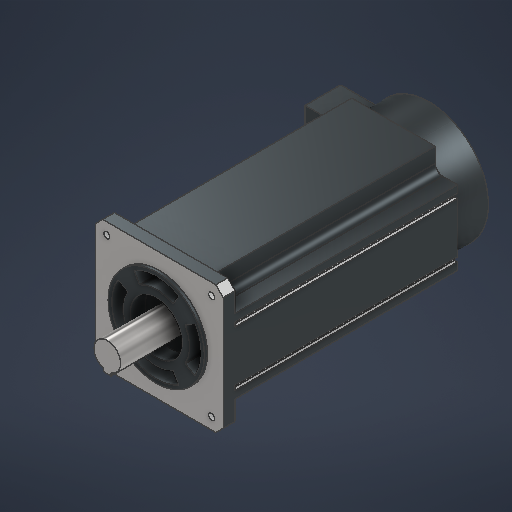
# Autodesk Inventor part: SERVOMOTOR-1KW
Saved by Autodesk Inventor 2025.3 (Build 293356030, 356C)
## iProperties
Created: 2025-09-01
Part Number: SERVOMOTOR-1KW
Material: Generic
Document SubType Name: Modeling
Designer: lstk1ng
Density: 1 g/cm^3
Appearance: Default
Author: lstk1ng
Autodesk Inventor part; units mm, degrees
ref_plane "YZ Plane" through (0, 0, 0) normal (1, 0, 0) x (0, 1, 0)
ref_plane "XZ Plane" through (0, 0, 0) normal (0, 1, 0) x (-1, 0, 0)
ref_plane "XY Plane" through (0, 0, 0) normal (0, 0, 1) x (1, 0, 0)
sketch "Sketch1" plane through (0, 0, 0) normal (0, 0, 1) x (1, 0, 0)
  line L0 (-38.15, 43.15) -> (38.15, 43.15)
  line L1 (43.15, 38.15) -> (43.15, -38.15)
  line L2 (38.15, -43.15) -> (-38.15, -43.15)
  line L3 (-43.15, -38.15) -> (-43.15, 38.15)
  circle A0 centre (0, 0) radius 32.5
  line L4 (-43.15, 38.15) -> (-38.15, 43.15)
  line L5 (38.15, 43.15) -> (43.15, 38.15)
  line L6 (-43.15, -38.15) -> (-38.15, -43.15)
  line L7 (38.15, -43.15) -> (43.15, -38.15)
  point P0 (-43.15, 43.15)
  point P1 (43.15, -43.15)
  point P2 (43.15, 43.15)
  point P3 (-43.15, -43.15)
  point P4 (-43.15, 0)
  dimension "d0" = 86.3
  dimension "d1" = 86.3
  dimension "d2" = 65
  dimension "d3" = 5
  dimension "d4" = 5
  dimension "d5" = 5
  dimension "d6" = 5
  dimension "d7" = 5
  dimension "d8" = 5
  dimension "d9" = 5
  dimension "d10" = 5
  constraints: 16 end point, 8 point on line, 2 parallel, 1 centre point, 1 coincident, 1 horizontal, 1 horizontal alignment, 1 midpoint, 1 perpendicular
  measures "d0" distance of point (43.15, -43.15) point (-43.15, -43.15)
  measures "d1" distance of point (43.15, 43.15) point (43.15, -43.15)
  measures "d2" diameter of A0
  measures "d3" distance of L3.end point (-43.15, 43.15)
  measures "d4" distance of L0.start point (-43.15, 43.15)
  measures "d5" distance of L0.end point (43.15, 43.15)
  measures "d6" distance of L1.start point (43.15, 43.15)
  measures "d7" distance of L3.start point (-43.15, -43.15)
  measures "d8" distance of L2.end point (-43.15, -43.15)
  measures "d9" distance of L2.start point (43.15, -43.15)
  measures "d10" distance of L1.end point (43.15, -43.15)
extrude "Extrusion1" add sketch "Sketch1" along normal blind 8
sketch "Sketch2" plane through (0, 0, 0) normal (0, 0, 1) x (1, 0, 0)
  circle A0 centre (0, 0) radius 32.5
  line L0 (11.25, 19.4856) -> (15, 25.9808)
  line L1 (0, 0) -> (30, 0) construction
  line L2 (-11.25, 19.4856) -> (-15, 25.9808)
  line L3 (0, 0) -> (30, 0) construction
  line L4 (-19.4856, -11.25) -> (-25.9808, -15)
  line L5 (-19.4856, 11.25) -> (-25.9808, 15)
  line L6 (11.25, -19.4856) -> (15, -25.9808)
  line L7 (-11.25, -19.4856) -> (-15, -25.9808)
  line L8 (19.4856, 11.25) -> (25.9808, 15)
  line L9 (19.4856, -11.25) -> (25.9808, -15)
  arc A1 (15, 25.9808) -> (-15, 25.9808) centre (0, 0) ccw
  arc A2 (25.9808, -15) -> (25.9808, 15) centre (0, 0) ccw
  arc A3 (-25.9808, 15) -> (-25.9808, -15) centre (0, 0) ccw
  arc A4 (-15, -25.9808) -> (15, -25.9808) centre (0, 0) ccw
  circle A5 centre (0, 0) radius 17.5
  arc A6 (-19.4856, 11.25) -> (-19.4856, -11.25) centre (0, 0) ccw
  arc A7 (-11.25, -19.4856) -> (11.25, -19.4856) centre (0, 0) ccw
  arc A8 (19.4856, -11.25) -> (19.4856, 11.25) centre (0, 0) ccw
  arc A9 (11.25, 19.4856) -> (-11.25, 19.4856) centre (0, 0) ccw
  dimension "d15" = 60
  dimension "d16" = 120
  dimension "d19" = 360
  dimension "d21" = 35
  constraints: 20 end point, 16 point on circle, 10 centre point, 4 coincident, 2 horizontal, 25 other
  measures "d15" angle of L1 L0
  measures "d16" angle of L3 L2
  measures "d21" diameter of A5
extrude "Extrusion2" add sketch "Sketch2" along normal blind 10
sketch "Sketch3" plane through (0, 0, 0) normal (0, 0, -1) x (-1, 0, 0)
  line L0 (-28.15, 40) -> (28.15, 40)
  line L1 (43.15, 25) -> (43.15, -25)
  line L2 (28.15, -40) -> (-28.15, -40)
  line L3 (-43.15, -25) -> (-43.15, 25)
  line L4 (-43.15, 40) -> (43.15, -40) construction
  line L5 (43.15, 40) -> (-43.15, -40) construction
  line L6 (-43.15, 25) -> (-28.15, 25)
  line L7 (-28.15, 25) -> (-28.15, 40)
  line L8 (28.15, 40) -> (28.15, 25)
  line L9 (28.15, 25) -> (43.15, 25)
  line L10 (-11.6946, 0) -> (10.241, 0) construction
  line L11 (-43.15, -25) -> (-28.15, -25)
  line L12 (-28.15, -25) -> (-28.15, -40)
  line L13 (28.15, -40) -> (28.15, -25)
  line L14 (28.15, -25) -> (43.15, -25)
  point P0 (0, 0)
  constraints: 30 end point, 6 symmetric about line, 3 perpendicular, 2 horizontal, 2 midpoint, 2 parallel
extrude "Extrusion3" add sketch "Sketch3" along normal blind 150
fillet "Fillet1" radius 5 4 edges at (28.15, 25, -75) (-28.15, 25, -75) (-28.15, -25, -75) (28.15, -25, -75)
sketch "Sketch4" plane through (0, 0, -150) normal (0, 0, -1) x (-1, 0, 0)
  arc A0 (34.641, 20) -> (34.641, -20) centre (0, 0) ccw
  line L0 (34.641, 20) -> (59.641, 20)
  line L1 (59.641, 20) -> (59.641, -20)
  line L2 (59.641, -20) -> (34.641, -20)
  dimension "d34" = 25
  dimension "d35" = 40
  constraints: 6 end point, 2 perpendicular, 2 point on circle, 1 centre point, 1 coincident, 1 horizontal
  measures "d34" distance of L0.start L0.end
  measures "d35" distance of L0.end L1.end
extrude "Extrusion4" add sketch "Sketch4" along normal blind 24
sketch "Sketch5" plane through (-43.15, -38.15, 8) normal (-1, 0, 0) x (0, 0, 1)
  line L0 (-158, 12.5091) -> (-158, 63.7909) projected
  line L1 (-158, 18.15) -> (-8, 18.15)
  line L2 (-8, 18.15) -> (-8, 21.15)
  line L3 (-8, 21.15) -> (-158, 21.15)
  line L4 (-158, 21.15) -> (-158, 18.15)
  line L5 (-8, 13.15) -> (-158, 13.15) projected
  line L6 (-158, 58.15) -> (-8, 58.15)
  line L7 (-8, 58.15) -> (-8, 55.15)
  line L8 (-8, 55.15) -> (-158, 55.15)
  line L9 (-158, 55.15) -> (-158, 58.15)
  line L10 (-8, 63.15) -> (-158, 63.15) projected
  point P0 (-8, 38.15)
  dimension "d38" = 3
  dimension "d39" = 5
  dimension "d40" = 3
  dimension "d41" = 5
  constraints: 16 end point, 4 parallel, 2 horizontal, 2 perpendicular, 2 point on line
  measures "d38" distance of L2.end L1.end
  measures "d39" distance between parallel lines of L5 L1
  measures "d40" distance of L6.end L7.end
  measures "d41" distance between parallel lines of L10 L6
extrude "Extrusion5" cut sketch "Sketch5" against normal blind 2
mirror "Mirror1" about plane through (0, 0, 0) normal (1, 0, 0) of "Extrusion5"
sketch "Sketch6" plane through (0, 0, 0) normal (0, 0, 1) x (1, 0, 0)
  arc A0 (2.5, -8.6458) -> (-2.5, -8.6458) centre (0, 0) ccw
  line L0 (0, -9) -> (0, -8) construction
  line L1 (0, -8) -> (-2.5, -8) construction
  line L2 (-2.5, -8) -> (0, -8) construction
  line L3 (2.5, -8) -> (2.5, -10.5)
  line L4 (2.5, -10.5) -> (-2.5, -10.5)
  line L5 (-2.5, -10.5) -> (-2.5, -8)
  dimension "d44" = 18
  dimension "d45" = 1
  dimension "d46" = 2.5
  dimension "d47" = 5
  dimension "d48" = 2.5
  constraints: 12 end point, 2 horizontal, 2 parallel, 2 point on circle, 2 point on line, 1 centre point, 1 coincident, 1 perpendicular, 1 vertical
  measures "d44" diameter of A0
  measures "d45" distance of L0.end L0.start
  measures "d46" distance of L0.end L1.end
  measures "d47" distance of L3.end L4.end
  measures "d48" distance of L3.start L3.end
extrude "Extrusion6" add sketch "Sketch6" along normal blind 43
sketch "Sketch7" plane through (0, 0, 8) normal (0, 0, 1) x (1, 0, 0)
  circle A0 centre (0, 0) radius 50 construction
  line L0 (-43.15, -43.15) -> (43.15, -43.15) construction
  line L1 (43.15, -43.15) -> (43.15, 43.15) construction
  line L2 (43.15, 43.15) -> (-43.15, 43.15) construction
  line L3 (-43.15, 43.15) -> (-43.15, -43.15) construction
  line L4 (-43.15, -43.15) -> (43.15, 43.15) construction
  line L5 (43.15, -43.15) -> (-43.15, 43.15) construction
  circle A1 centre (35.3553, 35.3553) radius 2.05
  circle A2 centre (35.3553, -35.3553) radius 2.05
  circle A3 centre (-35.3553, 35.3553) radius 2.05
  circle A4 centre (-35.3553, -35.3553) radius 2.05
  dimension "d51" = 100
  dimension "d52" = 4.1
  dimension "d53" = 4.1
  dimension "d54" = 4.1
  dimension "d55" = 4.1
  constraints: 12 end point, 5 centre point, 4 point on circle, 4 point on line, 2 midpoint, 2 parallel, 1 coincident, 1 horizontal, 1 perpendicular
  measures "d51" diameter of A0
  measures "d52" diameter of A1
  measures "d53" diameter of A2
  measures "d54" diameter of A3
  measures "d55" diameter of A4
extrude "Extrusion7" cut sketch "Sketch7" against normal up to surface (8 mm away)
equation "\"d4\" = d3"
equation "\"d5\" = d3"
equation "\"d6\" = d5"
equation "\"d7\" = d3"
equation "\"d8\" = d7"
equation "\"d9\" = d3"
equation "\"d10\" = d9"
equation "\"d56\" = d52"
body "Solid1"
